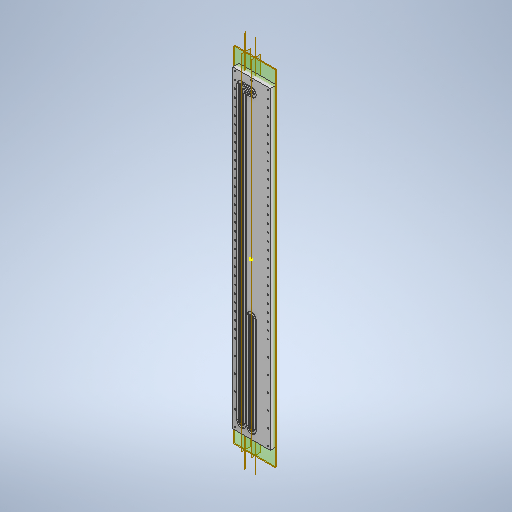
# Autodesk Inventor part: Bauteil5
Saved by Autodesk Inventor 2025 (Build 290162000, 162)
## iProperties
Created: 2024-12-16
Part Number: Bauteil5
Material: Generisch
Document SubType Name: Modeling
Designer: gorenfl4
Density: 1 g/cm^3
Appearance: Vorgabe
Author: gorenfl4
Autodesk Inventor part; units mm, degrees
ref_plane "YZ Plane" through (0, 0, 0) normal (1, 0, 0) x (0, 1, 0)
ref_plane "XZ Plane" through (0, 0, 0) normal (0, 1, 0) x (-1, 0, 0)
ref_plane "XY Plane" through (0, 0, 0) normal (0, 0, 1) x (1, 0, 0)
sketch "Skizze2" plane through (0, 0, 0) normal (0, 1, 0) x (-1, 0, 0)
  line L0 (30, 250) -> (-30, 250)
  line L1 (-30, 250) -> (-30, -250)
  line L2 (-30, -250) -> (30, -250)
  line L3 (30, -250) -> (30, 250)
  point P0 (0, 0)
  dimension "d21" = 500
  dimension "d22" = 60
  dimension "d23" = 30
  dimension "d24" = 250
  constraints: 8 end point, 2 parallel, 1 horizontal, 1 perpendicular
  measures "d21" distance of L2.end L0.start
  measures "d22" distance between parallel lines of L1 L3
  measures "d23" distance from line of point (0, 0) L1
  measures "d24" distance from line of L0 point (0, 0)
sketch "Skizze1" plane through (0, 0, 0) normal (0, 1, 0) x (-1, 0, 0)
  line L0 (22.5, 220) -> (22.5, -220)
  arc A0 (22.5, 220) -> (17.5, 225) centre (17.5, 220) ccw
  arc A1 (17.5, -225) -> (22.5, -220) centre (17.5, -220) ccw
  line L1 (17.5, 225) -> (-17.5, 225)
  line L2 (17.5, -225) -> (-17.5, -225)
  arc A2 (-17.5, 225) -> (-22.5, 220) centre (-17.5, 220) ccw
  arc A3 (-22.5, -220) -> (-17.5, -225) centre (-17.5, -220) ccw
  line L3 (-22.5, 220) -> (-22.5, -220)
  point P0 (0, 0)
  point P1 (0, 225)
  dimension "d0" = 90
  dimension "d1" = 5
  dimension "d3" = 22.5
  dimension "d4" = 5
  dimension "d5" = 90
  dimension "d13" = 35
  dimension "d14" = 35
  dimension "d15" = 5
  dimension "d16" = 90
  dimension "d17" = 5
  dimension "d18" = 90
  dimension "d19" = 45
  dimension "d285" = 225
  dimension "d286" = 450
  constraints: 9 point on circle, 8 end point, 4 centre point, 2 horizontal, 1 midpoint, 1 tangent, 1 vertical
  measures "d1" radius of A0
  measures "d3" distance from line of point (0, 0) L0
  measures "d4" radius of A1
  measures "d13" distance of L1.start L1.end
  measures "d14" distance of L2.start L2.end
  measures "d15" radius of A2
  measures "d17" radius of A3
  measures "d19" distance between parallel lines of L3 L0
  measures "d285" distance from line of L2 point (0, 0)
  measures "d286" distance between parallel lines of L2 L1
extrude "Extrusion1" add sketch "Skizze2" against normal blind 10
extrude "Extrusion2" cut sketch "Skizze1" against normal blind 1.6
sketch "Skizze6" plane through (0, -10, 0) normal (0, -1, 0) x (1, 0, 0)
  arc A0 (0, 228) -> (0, 232) centre (0, 230) ccw
  line L0 (-30, -250) -> (-30, 250) projected
  line L1 (-30, 250) -> (-30, -250) projected
  line L2 (0, 232) -> (-16, 232)
  arc A1 (-16, 232) -> (-18, 230) centre (-16, 230) ccw
  line L3 (-18, 230) -> (-18, -235)
  arc A2 (-18, -235) -> (-14, -235) centre (-16, -235) ccw
  line L4 (0, 228) -> (-14, 228)
  line L5 (-14, 228) -> (-14, -235)
  line L6 (-30, -250) -> (30, -250) projected
  line L7 (-17.5, -225) -> (17.5, -225) projected
  line L8 (30, 250) -> (-30, 250) projected
  point P0 (0, 0)
  dimension "d68" = 2
  dimension "d76" = 14
  dimension "d122" = 4
  dimension "d145" = 2
  dimension "d287" = 10
  dimension "d296" = 20
  constraints: 9 end point, 6 point on circle, 6 tangent, 3 centre point, 2 horizontal, 1 perpendicular, 1 vertical
  measures "d68" radius of A0
  measures "d76" distance from line of L0 A1.centre
  measures "d122" distance between parallel lines of L5 L3
  measures "d145" radius of A1
  measures "d287" distance from line of L7 A2.centre
  measures "d296" distance from line of L8 A0.centre
extrude "Extrusion4" cut sketch "Skizze6" against normal blind 1.9
sketch "Skizze13" plane through (0, -1.6, 0) normal (0, 1, 0) x (1, 0, 0)
  line L0 (-17.5, 225) -> (17.5, 225) projected
  line L1 (30, -250) -> (30, 250) projected
  point P0 (0, 0)
  point P1 (0, 80.9)
  dimension "d288" = 144.1
  dimension "d289" = 30
  measures "d288" distance from line of L0 point (0, 80.9)
  measures "d289" distance from line of L1 point (0, 80.9)
hole "Bohrung7" at (0, -1.6, -80.9) direction (0, -1, 0) diameter 4 end through all
sketch "Skizze7" plane through (0, -10, 0) normal (0, -1, 0) x (1, 0, 0)
  arc A0 (-2, -235) -> (0, -237) centre (0, -235) ccw
  line L0 (0, -237) -> (0, -237)
  arc A1 (0, -237) -> (2, -235) centre (0, -235) ccw
  line L1 (0, -235) -> (2, -235) construction
  line L2 (0, -235) -> (0, -237) construction
  circle A2 centre (0, -80.9) radius 2
  arc A3 (0, -78.9) -> (-2, -80.9) centre (0, -80.9) ccw
  line L3 (-2, -80.9) -> (-2, -235)
  line L4 (2, -235) -> (2, -80.9)
  line L5 (0, -78.9) -> (0, -78.9)
  arc A4 (2, -80.9) -> (0, -78.9) centre (0, -80.9) ccw
  arc A5 (-2, -235) -> (0, -237) centre (0, -235) ccw
  line L6 (3.5, -248.413) -> (3.5, -80.9)
  arc A6 (3.5, -80.9) -> (0, -77.4) centre (0, -80.9) ccw
  line L7 (0, -77.4) -> (0, -77.4)
  arc A7 (0, -77.4) -> (-3.5, -80.9) centre (0, -80.9) ccw
  line L8 (-3.5, -80.9) -> (-3.5, -248.413)
  line L9 (7, -248.413) -> (7, -80.9)
  arc A8 (7, -80.9) -> (0, -73.9) centre (0, -80.9) ccw
  line L10 (0, -73.9) -> (0, -73.9)
  arc A9 (0, -73.9) -> (-7, -80.9) centre (0, -80.9) ccw
  line L11 (-7, -80.9) -> (-7, -248.413)
  circle A10 centre (0, -80.9) radius 2 projected
  line L12 (-17.5, -225) -> (17.5, -225) projected
  point P0 (0, 0)
  point P1 (2, -80.9)
  point P2 (0, -237)
  dimension "d83" = 2
  dimension "d85" = 0
  dimension "d86" = 90
  dimension "d91" = 2
  dimension "d271" = 2
  dimension "d274" = 1.5
  dimension "d275" = 3.5
  dimension "d290" = 0
  dimension "d318" = 10
  constraints: 24 end point, 22 point on circle, 10 centre point, 7 tangent, 4 parallel, 2 horizontal, 2 vertical, 1 coincident, 4 other
  measures "d83" radius of A0
  measures "d85" distance of L0.start L0.end
  measures "d86" angle of L2 L1
  measures "d91" radius of A1
  measures "d271" radius of A4
  measures "d274" distance between parallel lines of L4 L6
  measures "d275" distance between parallel lines of L6 L9
  measures "d290" distance of A10.centre A3.centre
  measures "d318" distance from line of A0.centre L12
sketch "Skizze16" plane through (0, -8.1, 0) normal (0, -1, 0) x (1, 0, 0)
  arc A0 (-18, -235) -> (-14, -235) centre (-16, -235) ccw projected
  point P0 (0, 0)
  constraints: 1 coincident
hole "Bohrung10" at (-16, -8.1, -235) direction (0, 1, 0) diameter 4 depth 5 tip angle 118
sketch "Skizze18" plane through (0, -10, 0) normal (0, -1, 0) x (1, 0, 0)
  line L0 (-30, -250) -> (30, -250) projected
  line L1 (30, -250) -> (30, 250) projected
  point P0 (0, 0)
  point P1 (26.25, -246)
  dimension "d238" = 4
  dimension "d239" = 3.75
  measures "d238" distance from line of L0 point (26.25, -246)
  measures "d239" distance from line of L1 point (26.25, -246)
hole "Bohrung12" at (26.25, -10, -246) direction (0, 1, 0) diameter 2.013 end through all thread size "M2.5x0.45" class "6H" standard "ISO Metric profile"
pattern_linear "Rechteckige Anordnung5" count 11 spacing 49.2 along (0, 0, 1) count 2 spacing 52.5 along (-1, 0, 0) of "Bohrung12"
sketch "Skizze19" plane through (0, -10, 0) normal (0, -1, 0) x (1, 0, 0)
  circle A0 centre (0, 177.775) radius 2 projected
  arc A1 (0, 226.25) -> (0, 233.75) centre (0, 230) ccw
  arc A2 (-16, 233.75) -> (-19.75, 230) centre (-16, 230) ccw
  line L0 (0, 233.75) -> (-16, 233.75)
  arc A3 (-19.75, -235) -> (-12.25, -235) centre (-16, -235) ccw
  line L1 (-19.75, 230) -> (-19.75, -235)
  line L2 (0, 226.25) -> (-7.75, 226.25)
  line L3 (-12.25, -235) -> (-12.25, 221.75)
  arc A4 (-7.75, 226.25) -> (-12.25, 221.75) centre (-7.75, 221.75) ccw
  line L4 (0, 228) -> (-14, 228) projected
  arc A5 (0, 222.7) -> (0, 237.3) centre (0, 230) ccw
  line L5 (0, 222.7) -> (-7.75, 222.7)
  arc A6 (-7.75, 222.7) -> (-8.7, 221.75) centre (-7.75, 221.75) ccw
  line L6 (-8.7, 221.75) -> (-8.7, -235)
  arc A7 (-23.3, -235) -> (-8.7, -235) centre (-16, -235) ccw
  line L7 (-23.3, -235) -> (-23.3, 230)
  arc A8 (-16, 237.3) -> (-23.3, 230) centre (-16, 230) ccw
  line L8 (-16, 237.3) -> (0, 237.3)
  arc A9 (0, 228) -> (0, 232) centre (0, 230) ccw projected
  arc A10 (-16, 232) -> (-18, 230) centre (-16, 230) ccw projected
  line L9 (-17.5, -225) -> (17.5, -225) projected
  point P0 (0, 0)
  point P1 (0, 175.025)
  point P2 (0, 175.775)
  dimension "d253" = 3.75
  dimension "d254" = 3.75
  dimension "d255" = 3.75
  dimension "d256" = 1.75
  dimension "d258" = 4.5
  dimension "d259" = 4.5
  dimension "d260" = 3.55
  dimension "d319" = 10
  constraints: 16 end point, 16 point on circle, 8 centre point, 6 tangent, 2 concentric, 2 parallel, 1 horizontal, 1 vertical, 1 vertical alignment, 8 other
  measures "d253" radius of A1
  measures "d254" radius of A3
  measures "d255" radius of A2
  measures "d258" radius of A4
  measures "d259" distance from line of L3.end L2
  measures "d260" radial gap between concentric circles of A1 A5
  measures "d319" distance from line of L9 A3.centre
extrude "Extrusion8" cut sketch "Skizze7" against normal blind 1.9 contours L3 L12 L4 A1 A0 | L3 A2 L4 L12
sketch "Skizze21" plane through (0, -10, 0) normal (0, -1, 0) x (1, 0, 0)
  point P0 (0, 0)
sketch "Skizze22" plane through (0, -10, 0) normal (0, -1, 0) x (1, 0, 0)
  line L0 (3.75, -80.9) -> (3.75, -235)
  line L1 (2, -80.9) -> (2, -235) projected
  line L2 (-3.75, -80.9) -> (-3.75, -235)
  line L3 (-2, -235) -> (-2, -80.9) projected
  line L4 (0, -77.15) -> (0.0039, -77.15)
  line L5 (0, -238.75) -> (0, -238.75)
  arc A0 (-2, -235) -> (2, -235) centre (0, -235) ccw projected
  arc A1 (0, -238.75) -> (3.75, -235) centre (0, -235) ccw
  arc A2 (-3.75, -235) -> (0, -238.75) centre (0, -235) ccw
  arc A3 (3.75, -80.9) -> (0, -77.15) centre (0, -80.9) ccw
  arc A4 (3.5818, -79.7896) -> (-3.75, -80.9) centre (0, -80.9) ccw
  arc A5 (6.25, -77.1281) -> (-7.3, -80.9) centre (0, -80.9) ccw
  line L6 (-7.3, -80.9) -> (-7.3, -235)
  arc A6 (-7.3, -235) -> (0, -242.3) centre (0, -235) ccw
  line L7 (0, -242.3) -> (0, -242.3)
  arc A7 (0, -242.3) -> (7.3, -235) centre (0, -235) ccw
  line L8 (7.3, -235) -> (7.3, -80.9)
  arc A8 (7.3, -80.9) -> (0, -73.6) centre (0, -80.9) ccw
  line L9 (0, -73.6) -> (0.0039, -73.6)
  arc A9 (2, -80.9) -> (-2, -80.9) centre (0, -80.9) ccw projected
  line L10 (-2, -235) -> (-2, -80.9) projected
  arc A10 (2, -80.9) -> (-2, -80.9) centre (0, -80.9) ccw projected
  line L11 (2, -80.9) -> (2, -235) projected
  arc A11 (-2, -235) -> (2, -235) centre (0, -235) ccw projected
  circle A12 centre (-26.25, 246) radius 1.0065 projected
  circle A13 centre (-26.25, 196.8) radius 1.0065 projected
  circle A14 centre (-26.25, 147.6) radius 1.0065 projected
  circle A15 centre (-26.25, 98.4) radius 1.0065 projected
  circle A16 centre (-26.25, 49.2) radius 1.0065 projected
  circle A17 centre (-26.25, 0) radius 1.0065 projected
  circle A18 centre (-26.25, -49.2) radius 1.0065 projected
  circle A19 centre (-26.25, -98.4) radius 1.0065 projected
  circle A20 centre (-26.25, -147.6) radius 1.0065 projected
  circle A21 centre (-26.25, -196.8) radius 1.0065 projected
  circle A22 centre (-26.25, -246) radius 1.0065 projected
  circle A23 centre (26.25, 246) radius 1.0065 projected
  circle A24 centre (26.25, 196.8) radius 1.0065 projected
  circle A25 centre (26.25, 147.6) radius 1.0065 projected
  circle A26 centre (26.25, 98.4) radius 1.0065 projected
  circle A27 centre (26.25, 49.2) radius 1.0065 projected
  circle A28 centre (26.25, 0) radius 1.0065 projected
  circle A29 centre (26.25, -49.2) radius 1.0065 projected
  circle A30 centre (26.25, -98.4) radius 1.0065 projected
  circle A31 centre (26.25, -147.6) radius 1.0065 projected
  circle A32 centre (26.25, -196.8) radius 1.0065 projected
  circle A33 centre (26.25, -246) radius 1.0065 projected
  line L12 (-16, 232) -> (0, 232) projected
  arc A34 (0, 228) -> (0, 232) centre (0, 230) ccw projected
  line L13 (0, 228) -> (-14, 228) projected
  line L14 (-14, 228) -> (-14, -235) projected
  arc A35 (-18, -235) -> (-14, -235) centre (-16, -235) ccw projected
  line L15 (-18, -235) -> (-18, 230) projected
  arc A36 (-16, 232) -> (-18, 230) centre (-16, 230) ccw projected
  line L16 (30, -250) -> (30, 250) projected
  line L17 (30, 250) -> (-30, 250) projected
  line L18 (-30, 250) -> (-30, -250) projected
  line L19 (-30, -250) -> (30, -250) projected
  point P0 (0, 0)
  point P1 (0, -77.15)
  point P2 (0, -73.6)
  point P3 (0, -73.6)
  point P4 (0, -242.3)
  dimension "d276" = 1.75
  dimension "d277" = 1.75
  dimension "d292" = 3.55
  dimension "d295" = 3.75
  dimension "d329" = 3.75
  dimension "d382" = 1.75
  dimension "d384" = 1.75
  dimension "d385" = 7.3
  dimension "d386" = 7.3
  constraints: 16 end point, 16 point on circle, 10 tangent, 8 centre point, 2 coincident, 2 horizontal, 2 vertical, 4 other
  measures "d276" distance between parallel lines of L1 L0
  measures "d277" distance between parallel lines of L2 L3
  measures "d292" distance between parallel lines of L6 L2
  measures "d295" radius of A4
  measures "d329" radius of A3
  measures "d382" radial gap between concentric circles of A2 A0
  measures "d384" radial gap between concentric circles of A4 A9
  measures "d385" radius of A7
  measures "d386" radius of A6
extrude "Extrusion9" cut sketch "Skizze22" against normal blind 1.9 contours A8 L8 A7 A6 L6 A5
extrude "Extrusion10" cut sketch "Skizze19" against normal blind 1.9 contours L5 A6 L6 A7 L7 A8 L8 A5
sketch "Skizze23" plane through (0, -8.1, 0) normal (0, -1, 0) x (1, 0, 0)
  arc A0 (0, 228) -> (0, 232) centre (0, 230) ccw projected
  point P0 (0, 0)
  point P1 (0, 230)
  constraints: 1 coincident
hole "Bohrung13" at (0, -8.1, 230) direction (0, 1, 0) diameter 4 end through all
sketch "Skizze24" plane through (0, -1.6, 0) normal (0, 1, 0) x (1, 0, 0)
  line L0 (9, -200.6) -> (9, -214.6)
  line L1 (7, -216.6) -> (-7, -216.6)
  line L2 (-9, -214.6) -> (-9, -200.6)
  line L3 (-8.7, -221.75) -> (-8.7, 235) projected
  line L4 (-7, -198.6) -> (7, -198.6)
  arc A0 (7, -216.6) -> (9, -214.6) centre (7, -214.6) ccw
  arc A1 (-9, -214.6) -> (-7, -216.6) centre (-7, -214.6) ccw
  arc A2 (9, -200.6) -> (7, -198.6) centre (7, -200.6) ccw
  arc A3 (-7, -198.6) -> (-9, -200.6) centre (-7, -200.6) ccw
  line L5 (17.5, -225) -> (-17.5, -225) projected
  line L6 (22.5, 220) -> (22.5, -220) projected
  point P0 (0, 0)
  dimension "d304" = 18
  dimension "d305" = 18
  dimension "d306" = 2
  dimension "d307" = 2
  dimension "d308" = 2
  dimension "d309" = 2
  dimension "d310" = 8.4
  dimension "d312" = 9
  constraints: 8 end point, 8 point on circle, 8 tangent, 4 centre point, 2 horizontal, 1 parallel, 1 vertical
  measures "d304" distance between parallel lines of L4 L1
  measures "d305" distance between parallel lines of L2 L0
  measures "d306" radius of A0
  measures "d307" radius of A1
  measures "d308" radius of A2
  measures "d309" radius of A3
  measures "d310" distance between parallel lines of L5 L1
  measures "d312" distance from line of point (0, 0) L0
extrude "Extrusion11" add sketch "Skizze24" along normal blind 5.6
pattern_linear "Rechteckige Anordnung6" count 10 spacing 30 along (0, 0, -1) of "Extrusion11"
sketch "Skizze25" plane through (0, -8.1, 0) normal (0, -1, 0) x (1, 0, 0)
  arc A0 (-2, -235) -> (0, -237) centre (0, -235) ccw projected
  point P0 (0, 0)
  point P1 (0, -235)
  constraints: 1 coincident
hole "Bohrung14" at (0, -8.1, -235) direction (0, 1, 0) diameter 4 depth 5 tip angle 118
ref_plane "Arbeitsebene3" through (0, -5, 0) normal (0, 1, 0) x (1, 0, 0)
ref_plane "Arbeitsebene5" through (0, -3.5, 0) normal (0, 1, 0) x (1, 0, 0)
ref_plane "Arbeitsebene2" through (-16, -10, -235) normal (-1, 0, 0) x (0, 1, 0)
hole "Bohrung15" at (-16, -3.5, -250) direction (0, 0, 1) diameter 4.134 depth 14.2 tip angle 118 thread size "M5x0.8" class "6H" standard "ANSI Metric M Profile"
ref_plane "Arbeitsebene4" through (0, -10, -235) normal (-1, 0, 0) x (0, 1, 0)
hole "Bohrung16" at (0, -3.5, -250) direction (0, 0, 1) diameter 4.134 depth 14.2 tip angle 118 thread size "M5x0.8" class "6H" standard "ANSI Metric M Profile"
sketch "Skizze27" plane through (0, -1.6, 0) normal (0, 1, 0) x (1, 0, 0)
  point P0 (0, 0)
sketch "Skizze29" plane through (0, -1.6, 0) normal (0, 1, 0) x (1, 0, 0)
  line L0 (-17.5, 225) -> (17.5, 225) projected
  line L1 (-10.5, 225) -> (10.5, 225)
  line L2 (10.5, 225) -> (10.5, 100)
  line L3 (10.5, 100) -> (-10.5, 100)
  line L4 (-10.5, 100) -> (-10.5, 225)
  line L5 (-22.5, -220) -> (-22.5, 220) projected
  line L6 (22.5, 220) -> (22.5, -220) projected
  point P0 (0, 0)
  dimension "d375" = 125
  dimension "d376" = 12
  dimension "d377" = 12
  constraints: 8 end point, 2 parallel, 1 horizontal, 1 perpendicular, 1 point on line
  measures "d375" distance of L1.end L2.end
  measures "d376" distance between parallel lines of L5 L4
  measures "d377" distance between parallel lines of L6 L2
extrude "Extrusion12" cut sketch "Skizze29" against normal blind 3
fillet "Rundung1" radius 2 4 edges at (-10.5, -3.1, -100) (-10.5, -3.1, -225) (10.5, -3.1, -100) (10.5, -3.1, -225)
sketch "Skizze30" plane through (0, 0, 0) normal (0, 1, 0) x (1, 0, 0)
  line L0 (-30, -250) -> (30, -250) projected
  line L1 (-30, 250) -> (-30, -250) projected
  point P0 (0, 0)
  point P1 (0, -246.25)
  dimension "d387" = 3.75
  dimension "d388" = 30
  measures "d387" distance from line of L0 point (0, -246.25)
  measures "d388" distance from line of L1 point (0, -246.25)
hole "Bohrung19" at (0, 0, 246.25) direction (0, -1, 0) diameter 3 end through all
sketch "Skizze31" plane through (0, 0, 0) normal (0, 1, 0) x (1, 0, 0)
  line L0 (-30, -250) -> (30, -250) projected
  line L1 (-30, 250) -> (-30, -250) projected
  point P0 (0, 0)
  point P1 (-26.25, 110.7)
  dimension "d396" = 360.7
  dimension "d397" = 3.75
  measures "d396" distance from line of L0 point (-26.25, 110.7)
  measures "d397" distance from line of L1 point (-26.25, 110.7)
hole "Bohrung20" at (-26.25, 0, -110.7) direction (0, -1, 0) diameter 3 end through all
sketch "Skizze32" plane through (0, 0, 0) normal (0, 1, 0) x (1, 0, 0)
  line L0 (-30, -250) -> (30, -250) projected
  line L1 (30, -250) -> (30, 250) projected
  point P0 (0, 0)
  point P1 (26.25, -233.7)
  dimension "d409" = 16.3
  dimension "d410" = 3.75
  measures "d409" distance from line of L0 point (26.25, -233.7)
  measures "d410" distance from line of L1 point (26.25, -233.7)
hole "Bohrung Oberer Deckel" at (26.25, 0, 233.7) direction (0, -1, 0) diameter 2.459 end through all thread size "M3x0.5" class "6H" standard "ANSI Metric M Profile"
pattern_linear "Bohrungen Oberer Deckel" count 14 spacing 24.6 along (0, 0, -1) count 2 spacing 52.5 along (-1, 0, 0) of "Bohrung Oberer Deckel"
sketch "Skizze33" plane through (0, 0, 0) normal (0, 1, 0) x (1, 0, 0)
  line L0 (-30, -250) -> (30, -250) projected
  line L1 (30, -250) -> (30, 250) projected
  point P0 (0, 0)
  point P1 (26.25, -221.4)
  dimension "d424" = 28.6
  dimension "d425" = 3.75
  measures "d424" distance from line of L0 point (26.25, -221.4)
  measures "d425" distance from line of L1 point (26.25, -221.4)
hole "Bohrung Zentrierplatte" at (26.25, 0, 221.4) direction (0, -1, 0) diameter 2.459 end through all thread size "M3x0.5" class "6H" standard "ANSI Metric M Profile"
pattern_linear "Bohrung Zentrierokatte" count 10 spacing 49.2 along (0, 0, -1) count 2 spacing 52.5 along (-1, 0, 0) of "Bohrung Zentrierplatte"
